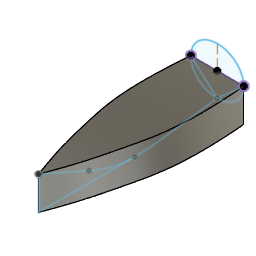
Robocon_Task2 (Autodesk Fusion 360 design; units mm, degrees)
Autodesk Fusion 360 part; units mm, degrees
sketch "Sketch1" plane through (0, 0, 0) normal (0, 0, 1) x (1, 0, 0)
  line L0 (-8, 4) -> (8, 4)
  line L1 (0, 0) -> (0, -50)
  spline S0 degree 5 poles (-8, 4) (-8.078, 3.0941) (-8.2223, 1.3102) (-8.4032, -1.2823) (-8.5734, -4.5714) (-8.6668, -8.4004) (-8.641, -11.9444) (-8.499, -15.2037) (-8.2479, -18.1844) (-7.9005, -20.9005) (-7.4782, -23.3784) (-7.0101, -25.6576) (-6.5248, -27.7849) (-6.0448, -29.8099) (-5.5788, -31.7809) (-5.1142, -33.7397) (-4.6247, -35.7232) (-4.08, -37.7655) (-3.4538, -39.8987) (-2.7341, -42.1556) (-1.9189, -44.5669) (-1.1938, -46.6403) (-0.6115, -48.2846) (-0.2066, -49.4214) (0, -50) knots 0 0 0 0 0 0 0.05 0.1 0.15 0.2 0.25 0.3 0.35 0.4 0.45 0.5 0.55 0.6 0.65 0.7 0.75 0.8 0.85 0.9 0.95 1 1 1 1 1 1
  line L2 (-2.1148, -44.0778) -> (2.1148, -55.9222)
  spline S1 degree 5 poles (8, 4) (8.077, 3.0973) (8.2194, 1.3191) (8.398, -1.2664) (8.5661, -4.5492) (8.6586, -8.3754) (8.6335, -11.9215) (8.4935, -15.1871) (8.2455, -18.1772) (7.9017, -20.904) (7.4824, -23.3912) (7.0156, -25.6747) (6.5294, -27.7987) (6.0457, -29.8125) (5.5743, -31.7672) (5.1054, -33.7131) (4.616, -35.6966) (4.0776, -37.7581) (3.4637, -39.9288) (2.7578, -42.228) (1.9512, -44.6653) (1.2227, -46.7285) (0.6295, -48.3396) (0.2133, -49.4418) (0, -50) knots 0 0 0 0 0 0 0.05 0.1 0.15 0.2 0.25 0.3 0.35 0.4 0.45 0.5 0.55 0.6 0.65 0.7 0.75 0.8 0.85 0.9 0.95 1 1 1 1 1 1
  point P0 (-8, -20)
  point P1 (-6, -30)
  point P2 (-4, -38)
  point P3 (8, -20)
  point P4 (6, -30)
  point P5 (4, -38)
  constraint horizontal L0
  constraint coincident L1.start origin
  constraint perpendicular L0 L1
  constraint midpoint L1.end L2
extrude "Extrude1" add sketch "Sketch1" along normal blind 10
sketch "Sketch2" plane through (0, 0, 0) normal (1, 0, 0) x (0, 1, 0)
  spline S0 degree 5 poles (-50, 10) (-49.3398, 9.7186) (-48.0239, 9.1545) (-46.064, 8.3051) (-43.4786, 7.1656) (-40.2935, 5.7365) (-37.1529, 4.3245) (-34.0513, 2.9728) (-30.977, 1.7569) (-27.9107, 0.7858) (-24.8147, 0.1554) (-21.6312, -0.0775) (-18.2603, 0.0419) (-14.5851, 0.3786) (-10.5539, 0.8681) (-6.1391, 1.4606) (-2.2969, 1.9994) (0.7577, 2.4355) (2.8704, 2.7405) (3.9458, 2.8965) knots 0 0 0 0 0 0 0.066667 0.133333 0.2 0.266667 0.333333 0.4 0.466667 0.533333 0.6 0.666667 0.733333 0.8 0.866667 0.933333 1 1 1 1 1 1
  line L0 (-25.9237, 0.0072) -> (-16, 0)
  line L1 (-50, 10) -> (-50, 0)
  line L2 (-50, 0) -> (-20.9618, 0.0036)
  line L3 (4, 10, 8) -> (3.9458, 2.8965, 0)
  line L4 (4, 10, -8) -> (3.9458, 2.8965, 0)
  curve E0
  line L5 (4.0542, 17.1035) -> (3.9458, 2.8965) construction
  line L6 (4, 10, -8) -> (4, 10, 8) construction
  line L7 (4, 10, 8) -> (4, 10, -8)
  point P0 (-34.781, 3.309)
  point P1 (-20.9618, 0.0036)
  point P2 (4, 10)
  point P3 (4, 10)
  constraint midpoint P1 L0
  constraint vertical L1
  constraint coincident P1 L2.end
  constraint coincident P3 P2
  constraint coincident S0.end L5.end
